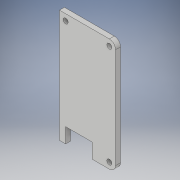
# Autodesk Inventor part: ScannerCover
Saved by Autodesk Inventor 2019 (Build 230136000, 136)
## iProperties
Created: 2019-01-25
Part Number: ScannerCover
Material: Generic
Document SubType Name: Modeling
Designer: garretthagen21
Density: 1 g/cm^3
Appearance: Default
Author: garretthagen21
Autodesk Inventor part; units mm, degrees
ref_plane "YZ Plane" through (0, 0, 0) normal (1, 0, 0) x (0, 1, 0)
ref_plane "XZ Plane" through (0, 0, 0) normal (0, 1, 0) x (-1, 0, 0)
ref_plane "XY Plane" through (0, 0, 0) normal (0, 0, 1) x (1, 0, 0)
sketch "Sketch1" plane through (0, 0, 0) normal (0, 0, 1) x (1, 0, 0)
  line L0 (-3.7023, -9.5266) -> (21.8247, -9.5266)
  line L1 (24.9997, -12.7016) -> (24.9997, -64.0096)
  line L2 (-3.7023, -67.1846) -> (-3.7023, -9.5266)
  line L3 (-0.5273, -67.1846) -> (-0.5273, -59.5646)
  line L4 (13.0617, -67.1846) -> (13.0617, -59.5646)
  line L5 (13.0617, -59.5646) -> (-0.5273, -59.5646)
  line L6 (21.8247, -67.1846) -> (13.0617, -67.1846)
  line L7 (-0.5273, -67.1846) -> (-3.7023, -67.1846)
  arc A0 (24.9997, -12.7016) -> (21.8247, -9.5266) centre (21.8247, -12.7016) ccw
  arc A1 (21.8247, -67.1846) -> (24.9997, -64.0096) centre (21.8247, -64.0096) ccw
  point P0 (0, 0)
  point P1 (24.9997, -67.1846)
  point P2 (24.9997, -9.5266)
  dimension "d1" = 57.658
  dimension "d3" = 7.62
  dimension "d11" = 11.938
  dimension "d12" = 28.702
  dimension "d21" = 7.62
  dimension "d23" = 3.175
  constraints: 16 end point, 4 point on circle, 4 point on line, 4 tangent, 3 parallel, 2 centre point, 2 perpendicular, 2 vertical, 1 equal radius, 1 horizontal
  measures "d1" distance of point (25, -9.527) point (25, -67.185)
  measures "d3" distance of L3.start L3.end
  measures "d11" distance between parallel lines of L1 L4
  measures "d12" distance between parallel lines of L1 L2
  measures "d21" distance of L4.start L4.end
  measures "d23" radius of A0
extrude "Scanner Cover" add sketch "Sketch1" along normal blind 2.54
sketch "Sketch2" plane through (0, 0, 2.54) normal (0, 0, 1) x (1, 0, 0)
  line L0 (-3.7023, -9.5266) -> (-3.7023, -67.1846) projected
  line L1 (21.8247, -9.5266) -> (-3.7023, -9.5266) projected
  line L2 (24.9997, -64.0096) -> (24.9997, -12.7016) projected
  line L3 (13.0617, -67.1846) -> (21.8247, -67.1846) projected
  point P0 (0, 0)
  point P1 (-0.5273, -12.7016)
  point P2 (24.9997, -9.5266)
  point P3 (21.8247, -12.7016)
  point P4 (24.9997, -67.1846)
  point P5 (21.8247, -64.0096)
  dimension "d7" = 3.175
  dimension "d8" = 3.175
  dimension "d9" = 3.175
  dimension "d10" = 3.175
  dimension "d13" = 3.175
  dimension "d22" = 3.175
  measures "d7" distance from line of L0 point (-0.527, -12.702)
  measures "d8" distance from line of L1 point (-0.527, -12.702)
  measures "d9" distance from line of point (21.825, -12.702) L1
  measures "d10" distance from line of point (21.825, -12.702) L2
  measures "d13" distance from line of point (21.825, -64.01) L3
  measures "d22" distance from line of L2 point (21.825, -64.01)
hole "Screw Holes" at (-0.5273, -12.7016, 2.54) at (21.8247, -12.7016, 2.54) at (21.8247, -64.0096, 2.54) direction (0, 0, -1) diameter 2.54 depth 25.4 tip angle 118
body "Solid1"
